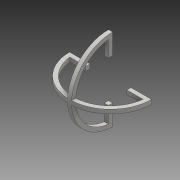
# Autodesk Inventor part: Bottom
Saved by Autodesk Inventor 2016 (Build 200138000, 138)
## iProperties
Created: 2015-12-29
Part Number: Bottom
Material: Generic
Document SubType Name: Modeling
Designer: Sudhar
Density: 1 g/cm^3
Appearance: Default
Author: Sudhar
Autodesk Inventor part; units mm, degrees
ref_plane "YZ Plane" through (0, 0, 0) normal (1, 0, 0) x (0, 1, 0)
ref_plane "XZ Plane" through (0, 0, 0) normal (0, 1, 0) x (-1, 0, 0)
ref_plane "XY Plane" through (0, 0, 0) normal (0, 0, 1) x (1, 0, 0)
sketch "Sketch1" plane through (0, 0, 0) normal (0, 0, 1) x (1, 0, 0)
  arc A0 (0, -50) -> (50, 0) centre (0, 0) ccw
  line L0 (0, 0) -> (0, -50)
  line L1 (0, 0) -> (50, 0)
  dimension "d0" = 100
  constraints: 4 end point, 2 point on circle, 1 centre point, 1 coincident, 1 perpendicular, 1 vertical
  measures "d0" diameter of A0
revolve "Revolution1" add sketch "Sketch1" angle 360 about axis through (0, 0, 0) along (0, -1, 0)
sketch "Sketch2" plane through (0, 0, 0) normal (0, 1, 0) x (1, 0, 0)
  line L0 (-49.9375, -2.5) -> (-2.5, -2.5)
  line L1 (2.5, -2.5) -> (49.9375, -2.5)
  line L2 (-2.5, 2.5) -> (-49.9375, 2.5)
  line L3 (49.9375, 2.5) -> (2.5, 2.5)
  line L4 (2.5, -49.9375) -> (2.5, -2.5)
  line L5 (2.5, 2.5) -> (2.5, 49.9375)
  line L6 (-2.5, 49.9375) -> (-2.5, 2.5)
  line L7 (-2.5, -2.5) -> (-2.5, -49.9375)
  arc A0 (2.3489, -49.9448) -> (49.9425, -2.3975) centre (0, 0) ccw
  arc A1 (49.9425, 2.3975) -> (2.3489, 49.9448) centre (0, 0) ccw
  arc A2 (-2.3489, 49.9448) -> (-49.9425, 2.3975) centre (0, 0) ccw
  arc A3 (-49.9425, -2.3975) -> (-2.3489, -49.9448) centre (0, 0) ccw
  point P0 (0, 0)
  constraints: 16 end point, 16 point on circle, 8 parallel, 4 centre point, 2 horizontal, 1 coincident
extrude "Extrusion1" cut sketch "Sketch2" against normal blind 100
shell "Shell1" thickness 5 removed faces 8 at (2.5, -32.793, -5.6262) at (-2.5, -32.793, -5.6262) at (-5.6262, -32.793, -2.5) at (-5.6262, -32.793, 2.5) at (-2.5, -32.793, 5.6262) at (2.5, -32.793, 5.6262) at (5.6262, -32.793, 2.5) at (5.6262, -32.793, -2.5)
sketch "Sketch3" plane through (-49.9375, 0, -2.5) normal (0, 1, 0) x (1, 0, 0)
  line L0 (24.9375, 22.5) -> (74.9375, 22.5)
  line L1 (74.9375, 22.5) -> (74.9375, -27.5)
  line L2 (74.9375, -27.5) -> (24.9375, -27.5)
  line L3 (24.9375, -27.5) -> (24.9375, 22.5)
  line L4 (24.9375, 22.5) -> (74.9375, -27.5) construction
  line L5 (74.9375, 22.5) -> (24.9375, -27.5) construction
  point P0 (49.9375, -2.5)
  dimension "d8" = 50
  dimension "d9" = 50
  constraints: 12 end point, 2 midpoint, 2 parallel, 1 horizontal, 1 perpendicular
  measures "d8" distance of L1.end L2.end
  measures "d9" distance of L2.end L0.start
extrude "Extrusion2" cut sketch "Sketch3" against normal blind 10
body "Solid1"
